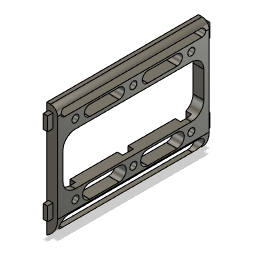
frontmount_a (Autodesk Fusion 360 design; units mm, degrees)
Autodesk Fusion 360 part; units mm, degrees
note: some values were not read from the file. Set by a fixed rule: which sketch regions a step uses.
sketch "Sketch1" plane through (0, 0, 0) normal (0, 0, 1) x (1, 0, 0)
  line L0 (0, 0) -> (0, 36)
  line L1 (0, 36) -> (2.4, 36)
  line L2 (2.4, 36) -> (2.4, 43.7)
  line L3 (2.4, 43.7) -> (0, 43.7)
  line L4 (0, 43.7) -> (0, 36)
  line L5 (0, 0) -> (2.4, 0)
  line L6 (2.4, 0) -> (2.4, -7.7)
  line L7 (2.4, -7.7) -> (0, -7.7)
  line L8 (0, -7.7) -> (0, 0)
  line L9 (5.042, 43.2) -> (5.042, -6.8)
  line L10 (0, 0) -> (0, -8)
  line L11 (0, -8) -> (-2.47, -8)
  line L12 (0, 36) -> (0, 44)
  line L13 (0, 43.7) -> (0, 47.2)
  line L14 (0, 47.2) -> (1.042, 47.2)
  line L15 (1.042, 47.2) -> (1.042, 43.2)
  arc A0 (5.042, 43.2) -> (1.042, 47.2) centre (1.042, 43.2) ccw
  line L16 (0, 47.2) -> (-1, 47.2)
  line L17 (-1, 47.2) -> (-1, -7.7)
  line L18 (-2.47, -8) -> (-2.47, -18.104)
  arc A1 (-2.47, -18.104) -> (5.042, -6.8) centre (-7.2191, -6.8) ccw
  line L19 (-1, -7.7) -> (-1, -17.3668)
  dimension "d1" = 36
  dimension "d2" = 2.4
  dimension "d3" = 7.7
  dimension "d4" = 2.4
  dimension "d5" = 7.7
  dimension "d9" = 50
  dimension "d11" = 8
  dimension "d12" = 2.47
  dimension "d14" = 8
  dimension "d15" = 3.5
  dimension "d16" = 1.042
  dimension "d17" = 4
  dimension "d18" = 1
  dimension "d19" = 10.104
  constraint coincident L0.start L5.start
  constraint vertical L0
  constraint horizontal L1
  constraint vertical L2
  constraint horizontal L3
  constraint vertical L4
  constraint horizontal L5
  constraint vertical L6
  constraint horizontal L7
  constraint vertical L8
  constraint vertical L9
  constraint perpendicular L5 L10
  constraint perpendicular L10 L11
  constraint perpendicular L1 L12
  constraint perpendicular L3 L13
  constraint perpendicular L13 L14
  constraint perpendicular L14 L15
  constraint coincident L15.end A0.centre
  constraint perpendicular L13 L16
  constraint perpendicular L7 L17
  constraint perpendicular L11 L18
  constraint tangent L9 A1
  constraint coincident A1 L19.end
  constraint perpendicular L11 L19
  measures "d1" distance of L0.start L0.end
  measures "d2" distance of L0.end L1.end
  measures "d3" distance of L0.end L3.end
  measures "d4" distance of L0.start L5.end
  measures "d5" distance of L0.start L7.end
  measures "d9" distance of L9.start L9.end
  measures "d11" distance of L0.start L10.end
  measures "d12" distance of L10.end L11.end
  measures "d14" distance of L0.end L12.end
  measures "d15" distance of L3.end L13.end
  measures "d16" distance of L13.end L14.end
  measures "d17" distance of L14.end L15.end
  measures "d18" distance of L13.end L16.end
  measures "d19" distance of L11.end L18.end
extrude "Extrude1" add sketch "Sketch1" against normal blind 3 contours L5 L6 L7 L8 L10 | L1 L2 L3 L4 L12 makes body 1 at (0, 41.1333, -1) makes body 2 at (2.4, -2.5667, -1)
extrude "Extrude2" add sketch "Sketch1" along normal blind 85 contours L0 L4 L8 L10 L11 L12 L13 L16 L17 L19 | L0 L1 L2 L3 L5 L6 L7 L9 L10 L11 L15 A0 A1 L19 | L5 L6 L7 L8 L10 | L1 L2 L3 L4 L12 | L3 L12 L13 L14 L15 bodies 1 2
sketch "Sketch2" plane through (0, 0, 85) normal (0, 0, 1) x (1, 0, 0)
  line L0 (1.042, 47.2) -> (-1, 47.2)
  line L1 (-1, 47.2) -> (-1, -17.3668)
  arc A0 (-1, -17.3668) -> (5.042, -6.8) centre (-7.2191, -6.8) ccw
  line L2 (5.042, -6.8) -> (5.042, 43.2)
  arc A1 (5.042, 43.2) -> (1.042, 47.2) centre (1.042, 43.2) ccw
  line L3 (-1, 47.2) -> (0, 47.2)
  line L4 (0, 47.2) -> (0, 43.7)
  line L5 (0, 43.7) -> (2.4, 43.7)
  line L6 (2.4, 43.7) -> (2.4, 36)
  line L7 (2.4, 36) -> (0, 36)
  line L8 (0, 36) -> (0, 43.7)
  line L9 (0, 0) -> (2.4, 0)
  line L10 (2.4, 0) -> (2.4, -7.7)
  line L11 (2.4, -7.7) -> (0, -7.7)
  line L12 (0, -7.7) -> (0, 0)
  dimension "d24" = 1
  dimension "d25" = 3.5
  dimension "d26" = 2.4
  dimension "d27" = 7.7
  dimension "d28" = 2.4
  dimension "d29" = 7.7
  constraint coincident L0.end L1.start
  constraint perpendicular L1 L3
  constraint perpendicular L0 L4
  constraint horizontal L5
  constraint vertical L6
  constraint horizontal L7
  constraint vertical L8
  constraint horizontal L9
  constraint vertical L10
  constraint horizontal L11
  constraint vertical L12
  constraint coincident L9.start L12.end
  measures "d24" distance of L0.end L3.end
  measures "d25" distance of L3.end L4.end
  measures "d26" distance of L4.end L5.end
  measures "d27" distance of L4.end L7.end
  measures "d28" distance of L9.start L9.end
  measures "d29" distance of L9.start L11.end
extrude "Extrude3" add sketch "Sketch2" along normal blind 3 contours L5 L6 L7 L8 | L9 L10 L11 L12 bodies 1
sketch "Sketch3" plane through (-1, 0, 0) normal (-1, 0, 0) x (0, 0, 1)
  line L0 (0, 47.2) -> (0, -17.3668)
  line L1 (0, -17.3668) -> (85, -17.3668)
  line L2 (85, -17.3668) -> (85, 47.2)
  line L3 (85, 47.2) -> (0, 47.2)
  line L4 (0, 47.2) -> (10, 47.2)
  line L5 (10, 47.2) -> (10, 32.2)
  line L6 (0, 47.2) -> (0, 25.2)
  line L7 (0, 25.2) -> (3, 25.2)
  line L8 (3, 25.2) -> (10, 25.2)
  arc A0 (10, 32.2) -> (3, 25.2) centre (10, 25.2) ccw
  line L9 (85, 47.2) -> (75, 47.2)
  line L10 (75, 47.2) -> (75, 32.2)
  line L11 (10, 32.2) -> (75, 32.2)
  line L12 (75, 32.2) -> (75, 25.2)
  arc A1 (81.9991, 25.3094) -> (75, 32.2) centre (75, 25.2) ccw
  line L13 (75, 25.2) -> (75, 10.2)
  arc A2 (75.0001, 3.2009) -> (81.9991, 10.2) centre (75, 10.2) ccw
  line L14 (10, 25.2) -> (10, 10.2)
  arc A3 (3, 10.2) -> (10, 3.2) centre (10, 10.2) ccw
  line L15 (3, 25.2) -> (3, 10.2)
  line L16 (10, 3.2) -> (75.0001, 3.2009)
  line L17 (81.9991, 10.2) -> (81.9991, 25.3094)
  dimension "d32" = 10
  dimension "d33" = 15
  dimension "d34" = 22
  dimension "d35" = 3
  dimension "d37" = 10
  dimension "d38" = 15
  dimension "d39" = 7
  dimension "d235" = 15
  dimension "d236" = 15
  constraint coincident L0.start L3.end
  constraint perpendicular L0 L4
  constraint perpendicular L3 L5
  constraint perpendicular L3 L6
  constraint perpendicular L6 L7
  constraint perpendicular L5 L8
  constraint coincident L8.end A0.centre
  constraint coincident L2.end L3.start
  constraint perpendicular L2 L9
  constraint perpendicular L3 L10
  constraint perpendicular L11 L12
  constraint coincident L12.end A1.centre
  constraint parallel L12 L13
  constraint coincident L13.end A2.centre
  constraint perpendicular L8 L14
  constraint coincident L14.end A3.centre
  constraint tangent A3 L15
  constraint tangent A2 L16
  constraint parallel L15 L17
  measures "d32" distance of L0.start L4.end
  measures "d33" distance of L4.end L5.end
  measures "d34" distance of L0.start L6.end
  measures "d35" distance of L6.end L7.end
  measures "d37" distance of L2.end L9.end
  measures "d38" distance of L9.end L10.end
  measures "d39" distance of L10.end L12.end
  measures "d235" distance of L12.end L13.end
  measures "d236" distance of L8.end L14.end
extrude "Extrude4" cut sketch "Sketch3" against normal blind 7 contours A0 L11 A1 A2 A3 L15 L16 L17 bodies 1
sketch "Sketch9" plane through (5.042, 0, 0) normal (1, 0, 0) x (0, 0, -1)
  line L0 (-75, 32.2) -> (-10, 32.2)
  arc A0 (-3, 25.2) -> (-10, 32.2) centre (-10, 25.2) ccw
  line L1 (-85, -6.8) -> (0, -6.8)
  line L2 (0, -6.8) -> (0, 43.2)
  line L3 (0, 43.2) -> (-85, 43.2)
  line L4 (-85, 43.2) -> (-85, -6.8)
  arc A1 (-75, 32.2) -> (-81.9991, 25.3094) centre (-75, 25.2) ccw
  line L5 (-74.9738, 2.9647) -> (-74.9738, -2.0353)
  line L6 (-75, 32.2) -> (-75, 37.2)
  line L7 (-9.9997, 3.2) -> (-9.9816, -1.8)
  line L8 (-42.4868, 3.0823) -> (-42.4686, -1.9176)
  line L9 (-10, 32.2) -> (-10, 37.2)
  line L10 (-42.5, 32.2) -> (-42.5, 37.2)
  circle A2 centre (-42.5, 37.2) radius 2
  circle A3 centre (-10, 37.2) radius 2
  circle A4 centre (-75, 37.2) radius 2
  circle A5 centre (-74.9738, -2.0353) radius 2
  circle A6 centre (-42.4686, -1.9176) radius 2
  circle A7 centre (-9.9816, -1.8) radius 2
  line L11 (-3, 25.2) -> (-3, 10.2)
  arc A8 (-10, 3.2) -> (-3, 10.2) centre (-10, 10.2) ccw
  line L12 (-10, 3.2) -> (-75.0001, 3.2009)
  arc A9 (-81.9991, 10.2) -> (-75.0001, 3.2009) centre (-75, 10.2) ccw
  line L13 (-81.9991, 10.2) -> (-81.9991, 25.3094)
  dimension "d151" = 5
  dimension "d152" = 5
  dimension "d153" = 5
  dimension "d154" = 5
  dimension "d155" = 5
  dimension "d156" = 5
  dimension "d157" = 4
  dimension "d158" = 4
  dimension "d159" = 4
  dimension "d160" = 4
  dimension "d161" = 4
  dimension "d162" = 4
  constraint coincident L0.start A1.start
  constraint perpendicular L1 L5
  constraint perpendicular L3 L6
  constraint coincident L0.end A0.end
  constraint perpendicular L0 L9
  constraint midpoint L0 L10.start
  constraint perpendicular L0 L10
  constraint coincident L10.end A2.centre
  constraint coincident L9.end A3.centre
  constraint coincident L6.end A4.centre
  constraint coincident L5.end A5.centre
  constraint coincident L8.end A6.centre
  constraint coincident L7.end A7.centre
  measures "d151" distance of L5.start L5.end
  measures "d152" distance of L0.start L6.end
  measures "d153" distance of L7.start L7.end
  measures "d154" distance of L8.start L8.end
  measures "d155" distance of L0.end L9.end
  measures "d156" distance of L10.start L10.end
  measures "d157" diameter of A2
  measures "d158" diameter of A3
  measures "d159" diameter of A4
  measures "d160" diameter of A5
  measures "d161" diameter of A6
  measures "d162" diameter of A7
extrude "Extrude18" cut sketch "Sketch9" against normal blind 20 contours A2 | A3 | A4 | A5 | A6 | A7 bodies 1
sketch "Sketch13" plane through (-1, 0, 0) normal (-1, 0, 0) x (0, 0, 1)
  circle A0 centre (10, 37.2) radius 2
  circle A1 centre (74.9738, -2.0353) radius 2
  circle A2 centre (42.5, 37.2) radius 2
  circle A3 centre (9.9816, -1.8) radius 2
  circle A4 centre (42.4686, -1.9176) radius 2
  circle A5 centre (75, 37.2) radius 2
  arc A6 (10, 32.2) -> (3, 25.2) centre (10, 25.2) ccw
  line L0 (10, 32.2) -> (75, 32.2)
  arc A7 (81.9991, 25.3094) -> (75, 32.2) centre (75, 25.2) ccw
  line L1 (0, 47.2) -> (0, -17.3668)
  line L2 (0, -17.3668) -> (85, -17.3668)
  line L3 (85, -17.3668) -> (85, 47.2)
  line L4 (85, 47.2) -> (0, 47.2)
  circle A8 centre (74.9738, -2.0353) radius 3
  circle A9 centre (42.4686, -1.9176) radius 3
  circle A10 centre (9.9816, -1.8) radius 3
  circle A11 centre (10, 37.2) radius 3
  circle A12 centre (42.5, 37.2) radius 3
  circle A13 centre (75, 37.2) radius 3
  line L5 (78, 37.2) -> (78, 31.5246)
  line L6 (72, 37.2) -> (72, 32.2)
  line L7 (45.5, 37.2) -> (45.5, 32.2)
  line L8 (39.5, 37.2) -> (39.5, 32.2)
  line L9 (13, 37.2) -> (13, 32.2)
  line L10 (7, 37.2) -> (7, 31.5246)
  line L11 (3, 10.2) -> (3, 25.2)
  line L12 (81.9991, 25.3094) -> (81.9991, 10.2)
  arc A14 (75.0001, 3.2009) -> (81.9991, 10.2) centre (75, 10.2) ccw
  line L13 (75.0001, 3.2009) -> (10, 3.2)
  arc A15 (3, 10.2) -> (10, 3.2) centre (10, 10.2) ccw
  line L14 (6.9816, -1.8) -> (6.9816, 3.8842)
  line L15 (12.9816, -1.8) -> (12.9816, 3.2)
  line L16 (39.4686, -1.9176) -> (39.4686, 3.2004)
  line L17 (45.4686, -1.9176) -> (45.4686, 3.2005)
  line L18 (71.9738, -2.0353) -> (71.9738, 3.2008)
  line L19 (77.9738, -2.0353) -> (77.9738, 3.864)
  dimension "d163" = 6
  dimension "d164" = 6
  dimension "d165" = 6
  dimension "d166" = 6
  dimension "d167" = 6
  dimension "d168" = 6
  constraint concentric A1 A8
  constraint concentric A4 A9
  constraint concentric A3 A10
  constraint concentric A0 A11
  constraint concentric A2 A12
  constraint concentric A5 A13
  constraint coincident A13 L5.start
  constraint coincident A7 L5.end
  constraint tangent A13 L5
  constraint vertical L5
  constraint coincident A13 L6.start
  constraint coincident L0 L6.end
  constraint tangent A13 L6
  constraint perpendicular L0 L6
  constraint coincident A12 L7.start
  constraint coincident L0 L7.end
  constraint tangent A12 L7
  constraint perpendicular L0 L7
  constraint coincident A12 L8.start
  constraint coincident L0 L8.end
  constraint tangent A12 L8
  constraint perpendicular L0 L8
  constraint coincident A11 L9.start
  constraint coincident L0 L9.end
  constraint tangent A11 L9
  constraint perpendicular L0 L9
  constraint coincident A11 L10.start
  constraint coincident A6 L10.end
  constraint tangent A11 L10
  constraint perpendicular L0 L10
  constraint coincident A10 L14.start
  constraint coincident A15 L14.end
  constraint tangent A10 L14
  constraint vertical L14
  constraint coincident A10 L15.start
  constraint coincident L13 L15.end
  constraint tangent A10 L15
  constraint vertical L15
  constraint coincident A9 L16.start
  constraint coincident L13 L16.end
  constraint tangent A9 L16
  constraint vertical L16
  constraint coincident A9 L17.start
  constraint coincident L13 L17.end
  constraint tangent A9 L17
  constraint parallel L16 L17
  constraint coincident A8 L18.start
  constraint coincident L13 L18.end
  constraint tangent A8 L18
  constraint parallel L17 L18
  constraint coincident A8 L19.start
  constraint coincident A14 L19.end
  constraint tangent A8 L19
  constraint parallel L18 L19
  measures "d163" diameter of A8
  measures "d164" diameter of A9
  measures "d165" diameter of A10
  measures "d166" diameter of A11
  measures "d167" diameter of A12
  measures "d168" diameter of A13
extrude "Extrude23" cut sketch "Sketch13" against normal blind 3 contours A6 L0 A11 L9 L10 | A11 | L0 A12 L7 L8 | A12 | A10 L13 A15 L14 L15 | L0 A7 A13 L5 L6 | A10 | A13 | A9 L13 L16 L17 | A9 | A8 A14 L13 L18 L19 | A8 bodies 1
sketch "Sketch14" plane through (-1, 0, 0) normal (-1, 0, 0) x (0, 0, 1)
  line L0 (0, 47.2) -> (0, -17.3668)
  line L1 (0, -17.3668) -> (85, -17.3668)
  line L2 (85, -17.3668) -> (85, 47.2)
  line L3 (85, 47.2) -> (0, 47.2)
  arc A0 (7, 31.5246) -> (3, 25.2) centre (10, 25.2) ccw
  line L4 (7, 31.5246) -> (7, 37.2)
  arc A1 (13, 37.2) -> (7, 37.2) centre (10, 37.2) ccw
  line L5 (13, 37.2) -> (13, 32.2)
  line L6 (13, 32.2) -> (39.5, 32.2)
  line L7 (39.5, 32.2) -> (39.5, 37.2)
  arc A2 (45.5, 37.2) -> (39.5, 37.2) centre (42.5, 37.2) ccw
  line L8 (45.5, 37.2) -> (45.5, 32.2)
  line L9 (45.5, 32.2) -> (72, 32.2)
  line L10 (72, 32.2) -> (72, 37.2)
  arc A3 (78, 37.2) -> (72, 37.2) centre (75, 37.2) ccw
  line L11 (78, 37.2) -> (78, 31.5246)
  arc A4 (81.9991, 25.3094) -> (78, 31.5246) centre (75, 25.2) ccw
  line L12 (0, -11.3668) -> (6, -11.3668)
  line L13 (85, -11.3668) -> (79, -11.3668)
  circle A5 centre (6, -11.3668) radius 4
  circle A6 centre (79, -11.3668) radius 4
  line L14 (79, -7.3668) -> (6, -7.3668)
  line L15 (6, -15.3668) -> (79, -15.3668)
  line L16 (81.9991, 25.3094) -> (81.9991, 10.2)
  arc A7 (77.9738, 3.864) -> (81.9991, 10.2) centre (75, 10.2) ccw
  line L17 (71.9738, 3.2008) -> (45.4686, 3.2005)
  arc A8 (3, 10.2) -> (6.9816, 3.8842) centre (10, 10.2) ccw
  line L18 (3, 10.2) -> (3, 25.2)
  line L19 (77.9738, 3.864) -> (77.9738, -2.0353)
  arc A9 (71.9738, -2.0353) -> (77.9738, -2.0353) centre (74.9738, -2.0353) ccw
  line L20 (71.9738, -2.0353) -> (71.9738, 3.2008)
  line L21 (45.4686, 3.2005) -> (45.4686, -1.9176)
  arc A10 (39.4686, -1.9176) -> (45.4686, -1.9176) centre (42.4686, -1.9176) ccw
  line L22 (39.4686, -1.9176) -> (39.4686, 3.2004)
  line L23 (39.4686, 3.2004) -> (12.9816, 3.2)
  line L24 (12.9816, 3.2) -> (12.9816, -1.8)
  arc A11 (6.9816, -1.8) -> (12.9816, -1.8) centre (9.9816, -1.8) ccw
  line L25 (6.9816, -1.8) -> (6.9816, 3.8842)
  dimension "d224" = 6
  dimension "d225" = 6
  dimension "d226" = 8
  dimension "d227" = 8
  constraint coincident L0 L12.start
  constraint perpendicular L0 L12
  constraint coincident L2 L13.start
  constraint perpendicular L2 L13
  constraint coincident L12.end A5.centre
  constraint coincident L13.end A6.centre
  constraint coincident A6 L14.start
  constraint coincident A5 L14.end
  constraint tangent A5 L14
  constraint parallel L13 L14
  constraint coincident A5 L15.start
  constraint coincident A6 L15.end
  constraint tangent A6 L15
  constraint parallel L12 L15
  measures "d224" distance of L12.start L12.end
  measures "d225" distance of L13.start L13.end
  measures "d226" diameter of A5
  measures "d227" diameter of A6
extrude "Extrude24" cut sketch "Sketch14" against normal blind 8 contours A5 | A5 A6 L14 L15 | A6 bodies 1
sketch "Sketch15" plane through (-1, 0, 0) normal (-1, 0, 0) x (0, 0, 1)
  line L0 (0, 47.2) -> (0, -17.3668)
  line L1 (0, -17.3668) -> (85, -17.3668)
  line L2 (85, -17.3668) -> (85, 47.2)
  line L3 (85, 47.2) -> (0, 47.2)
  arc A0 (7, 31.5246) -> (3, 25.2) centre (10, 25.2) ccw
  line L4 (7, 31.5246) -> (7, 37.2)
  arc A1 (13, 37.2) -> (7, 37.2) centre (10, 37.2) ccw
  line L5 (13, 37.2) -> (13, 32.2)
  line L6 (13, 32.2) -> (39.5, 32.2)
  line L7 (39.5, 32.2) -> (39.5, 37.2)
  arc A2 (45.5, 37.2) -> (39.5, 37.2) centre (42.5, 37.2) ccw
  line L8 (45.5, 37.2) -> (45.5, 32.2)
  line L9 (45.5, 32.2) -> (72, 32.2)
  line L10 (72, 32.2) -> (72, 37.2)
  arc A3 (78, 37.2) -> (72, 37.2) centre (75, 37.2) ccw
  line L11 (78, 37.2) -> (78, 31.5246)
  arc A4 (81.9991, 25.3094) -> (78, 31.5246) centre (75, 25.2) ccw
  arc A5 (79, -15.3668) -> (79, -7.3668) centre (79, -11.3668) ccw
  line L12 (79, -15.3668) -> (6, -15.3668)
  arc A6 (6, -7.3668) -> (6, -15.3668) centre (6, -11.3668) ccw
  line L13 (6, -7.3668) -> (79, -7.3668)
  line L14 (85, 43.2) -> (81, 43.2)
  line L15 (81.9991, 25.3094) -> (81.9991, 10.2)
  arc A7 (77.9738, 3.864) -> (81.9991, 10.2) centre (75, 10.2) ccw
  line L16 (71.9738, 3.2008) -> (45.4686, 3.2005)
  arc A8 (3, 10.2) -> (6.9816, 3.8842) centre (10, 10.2) ccw
  line L17 (3, 10.2) -> (3, 25.2)
  line L18 (0, 43.2569) -> (4, 43.2569)
  circle A9 centre (4, 43.2569) radius 2
  circle A10 centre (81, 43.2) radius 2
  line L19 (81, 45.2) -> (4.0015, 45.2569)
  line L20 (4, 41.2569) -> (80.9985, 41.2)
  line L21 (77.9738, 3.864) -> (77.9738, -2.0353)
  arc A11 (71.9738, -2.0353) -> (77.9738, -2.0353) centre (74.9738, -2.0353) ccw
  line L22 (71.9738, -2.0353) -> (71.9738, 3.2008)
  line L23 (45.4686, 3.2005) -> (45.4686, -1.9176)
  arc A12 (39.4686, -1.9176) -> (45.4686, -1.9176) centre (42.4686, -1.9176) ccw
  line L24 (39.4686, -1.9176) -> (39.4686, 3.2004)
  line L25 (39.4686, 3.2004) -> (12.9816, 3.2)
  line L26 (12.9816, 3.2) -> (12.9816, -1.8)
  arc A13 (6.9816, -1.8) -> (12.9816, -1.8) centre (9.9816, -1.8) ccw
  line L27 (6.9816, -1.8) -> (6.9816, 3.8842)
  dimension "d232" = 4
  dimension "d237" = 4
  dimension "d238" = 4
  dimension "d239" = 4
  constraint coincident L2 L14.start
  constraint perpendicular L2 L14
  constraint coincident L0 L18.start
  constraint perpendicular L0 L18
  constraint coincident L18.end A9.centre
  constraint coincident L14.end A10.centre
  constraint coincident A10 L19.start
  constraint coincident A9 L19.end
  constraint tangent A9 L19
  constraint coincident A9 L20.start
  constraint coincident A10 L20.end
  constraint tangent A10 L20
  constraint parallel L19 L20
  measures "d232" distance of L14.start L14.end
  measures "d237" distance of L18.start L18.end
  measures "d238" diameter of A9
  measures "d239" diameter of A10
extrude "Extrude25" cut sketch "Sketch15" against normal blind 10 contours A9 | A9 A10 L19 L20 | A10 bodies 1
sketch "Sketch16" plane through (-1, 0, 0) normal (-1, 0, 0) x (0, 0, 1)
  line L0 (0, 47.2) -> (0, -17.3668)
  line L1 (0, -17.3668) -> (85, -17.3668)
  line L2 (85, -17.3668) -> (85, 47.2)
  line L3 (85, 47.2) -> (0, 47.2)
  arc A0 (7, 31.5246) -> (3, 25.2) centre (10, 25.2) ccw
  line L4 (7, 31.5246) -> (7, 37.2)
  arc A1 (13, 37.2) -> (7, 37.2) centre (10, 37.2) ccw
  line L5 (13, 37.2) -> (13, 32.2)
  line L6 (13, 32.2) -> (39.5, 32.2)
  line L7 (39.5, 32.2) -> (39.5, 37.2)
  arc A2 (45.5, 37.2) -> (39.5, 37.2) centre (42.5, 37.2) ccw
  line L8 (45.5, 37.2) -> (45.5, 32.2)
  line L9 (45.5, 32.2) -> (72, 32.2)
  line L10 (72, 32.2) -> (72, 37.2)
  arc A3 (78, 37.2) -> (72, 37.2) centre (75, 37.2) ccw
  line L11 (78, 37.2) -> (78, 31.5246)
  arc A4 (81.9991, 25.3094) -> (78, 31.5246) centre (75, 25.2) ccw
  line L12 (10, 37.2) -> (18, 37.2)
  line L13 (75, 37.2) -> (67, 37.2)
  line L14 (42.5, 37.2) -> (50.5, 37.2)
  line L15 (42.5, 37.2) -> (34.5, 37.2)
  circle A5 centre (18, 37.2) radius 3
  circle A6 centre (34.5, 37.2) radius 3
  circle A7 centre (50.5, 37.2) radius 3
  circle A8 centre (67, 37.2) radius 3
  line L16 (50.5, 34.2) -> (67, 34.2)
  line L17 (67, 40.2) -> (50.5, 40.2)
  line L18 (34.5, 40.2) -> (18, 40.2)
  line L19 (18, 34.2) -> (34.5, 34.2)
  arc A9 (79, -15.3668) -> (79, -7.3668) centre (79, -11.3668) ccw
  line L20 (79, -15.3668) -> (6, -15.3668)
  arc A10 (6, -7.3668) -> (6, -15.3668) centre (6, -11.3668) ccw
  line L21 (6, -7.3668) -> (79, -7.3668)
  line L22 (81.9991, 25.3094) -> (81.9991, 10.2)
  arc A11 (77.9738, 3.864) -> (81.9991, 10.2) centre (75, 10.2) ccw
  line L23 (71.9738, 3.2008) -> (45.4686, 3.2005)
  arc A12 (3, 10.2) -> (6.9816, 3.8842) centre (10, 10.2) ccw
  line L24 (3, 10.2) -> (3, 25.2)
  arc A13 (80.9985, 41.2) -> (81, 45.2) centre (81, 43.2) ccw
  line L25 (80.9985, 41.2) -> (4, 41.2569)
  arc A14 (4.0015, 45.2569) -> (4, 41.2569) centre (4, 43.2569) ccw
  line L26 (4.0015, 45.2569) -> (81, 45.2)
  line L27 (77.9738, 3.864) -> (77.9738, -2.0353)
  arc A15 (71.9738, -2.0353) -> (77.9738, -2.0353) centre (74.9738, -2.0353) ccw
  line L28 (71.9738, -2.0353) -> (71.9738, 3.2008)
  line L29 (45.4686, 3.2005) -> (45.4686, -1.9176)
  arc A16 (39.4686, -1.9176) -> (45.4686, -1.9176) centre (42.4686, -1.9176) ccw
  line L30 (39.4686, -1.9176) -> (39.4686, 3.2004)
  line L31 (39.4686, 3.2004) -> (12.9816, 3.2)
  line L32 (12.9816, 3.2) -> (12.9816, -1.8)
  arc A17 (6.9816, -1.8) -> (12.9816, -1.8) centre (9.9816, -1.8) ccw
  line L33 (6.9816, -1.8) -> (6.9816, 3.8842)
  line L34 (42.4686, -1.9176) -> (34.4686, -1.9176)
  line L35 (34.4686, -1.9176) -> (17.9686, -1.9176)
  circle A18 centre (34.4686, -1.9176) radius 4
  circle A19 centre (17.9686, -1.9176) radius 4
  line L36 (42.4686, -1.9176) -> (50.4686, -1.9176)
  line L37 (50.4686, -1.9176) -> (66.9686, -1.9176)
  circle A20 centre (50.4686, -1.9176) radius 4
  circle A21 centre (66.9686, -1.9176) radius 4
  line L38 (17.9686, 2.0824) -> (34.4686, 2.0824)
  line L39 (34.4686, -5.9176) -> (17.9686, -5.9176)
  line L40 (50.4686, -5.9176) -> (66.9686, -5.9176)
  line L41 (66.9686, 2.0824) -> (50.4686, 2.0824)
  dimension "d207" = 8
  dimension "d208" = 8
  dimension "d209" = 8
  dimension "d210" = 8
  dimension "d211" = 6
  dimension "d212" = 6
  dimension "d213" = 6
  dimension "d214" = 6
  dimension "d242" = 8
  dimension "d243" = 16.5
  dimension "d244" = 8
  dimension "d245" = 8
  dimension "d246" = 8
  dimension "d247" = 16.5
  dimension "d248" = 8
  dimension "d249" = 8
  constraint horizontal L13
  constraint coincident L12.end A5.centre
  constraint coincident L15.end A6.centre
  constraint coincident L14.end A7.centre
  constraint coincident L13.end A8.centre
  constraint coincident A7 L16.start
  constraint coincident A8 L16.end
  constraint tangent A8 L16
  constraint horizontal L16
  constraint coincident A8 L17.start
  constraint coincident A7 L17.end
  constraint tangent A7 L17
  constraint horizontal L17
  constraint coincident A6 L18.start
  constraint coincident A5 L18.end
  constraint tangent A5 L18
  constraint parallel L17 L18
  constraint coincident A5 L19.start
  constraint coincident A6 L19.end
  constraint tangent A6 L19
  constraint parallel L18 L19
  constraint coincident A2.centre L14.start
  constraint coincident A3.centre L13.start
  constraint coincident A16.centre L34.start
  constraint horizontal L34
  constraint parallel L34 L35
  constraint coincident L34.end L35.start
  constraint coincident L35.end A19.centre
  constraint parallel L34 L36
  constraint parallel L36 L37
  constraint coincident L36.end L37.start
  constraint coincident L37.end A21.centre
  constraint coincident A19 L38.start
  constraint coincident A18 L38.end
  constraint tangent A18 L38
  constraint parallel L35 L38
  constraint coincident A18 L39.start
  constraint coincident A19 L39.end
  constraint tangent A19 L39
  constraint parallel L35 L39
  constraint coincident A20 L40.start
  constraint coincident A21 L40.end
  constraint tangent A21 L40
  constraint parallel L39 L40
  constraint coincident A21 L41.start
  constraint coincident A20 L41.end
  constraint tangent A20 L41
  constraint parallel L40 L41
  measures "d207" distance of A1.centre L12.end
  measures "d208" distance of A3.centre L13.end
  measures "d209" distance of A2.centre L14.end
  measures "d210" distance of A2.centre L15.end
  measures "d211" diameter of A5
  measures "d212" diameter of A6
  measures "d213" diameter of A7
  measures "d214" diameter of A8
  measures "d242" distance of A16.centre L34.end
  measures "d243" distance of L34.end L35.end
  measures "d244" diameter of A18
  measures "d245" diameter of A19
  measures "d246" distance of A16.centre L36.end
  measures "d247" distance of L36.end L37.end
  measures "d248" diameter of A20
  measures "d249" diameter of A21
extrude "Extrude26" cut sketch "Sketch16" against normal blind 8.5 contours A5 | A5 A6 L18 L19 | A6 | A7 | A7 A8 L16 L17 | A8 | L34 L35 A18 | L34 L35 A18 | L35 A18 A19 L38 | L35 A18 A19 L39 | A19 | L36 L37 A20 | L36 L37 A20 | L37 A20 A21 L41 | L37 A20 A21 L40 | A21 bodies 1
